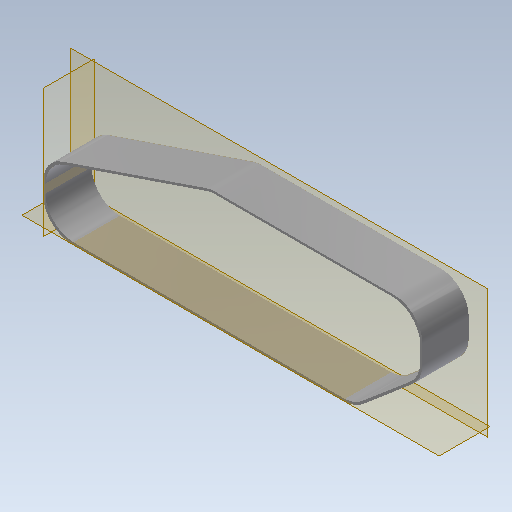
# Autodesk Inventor part: Rupsband
Saved by Autodesk Inventor 2021 (Build 250183000, 183)
## iProperties
Manager: PJ / DCS
Company: Emmaüs Bovenbouw Aalter
Created: 2020-11-19
Part Number: Rupsband
Material: S235
Catalog Web Link: http://emmausbovenbouw.op-weg.be/
Vendor: Emmaüsinstituut Bovenbouw Aalter
Document SubType Name: Modeling
Designer: Antho
Engineer: Declercq St.
Manufacturer: Standard
Standards Organization: Custom
Density: 7.86 g/cm^3
Appearance: Steel
Title: Algemene titel
Subject: Specifieke titel
Author: Antho
Keywords: Ruwe Ø xxxxx
Comments: Opmerking
Autodesk Inventor part; units mm, degrees
sketch "Sketch3" plane through (0, 0, 0) normal (0, 0, 1) x (1, 0, 0)
  line L0 (0, 0) -> (0, 51)
  line L1 (0, 51) -> (150, 51)
  line L2 (150, 51) -> (150, 102)
  line L3 (150, 102) -> (340, 102)
  line L4 (340, 102) -> (340, 51)
  line L5 (340, 51) -> (280, 51)
  line L6 (280, 51) -> (280, 0)
  line L7 (280, 0) -> (0, 0)
  line L8 (0, 51) -> (150, 102)
  line L9 (280, 0) -> (340, 51)
  dimension "d9" = 51
  dimension "d10" = 150
  dimension "d11" = 51
  dimension "d12" = 190
  dimension "d13" = 51
  dimension "d14" = 60
  constraints: 20 end point, 5 perpendicular, 2 point on line, 1 vertical
  measures "d9" distance of L0.start L0.end
  measures "d10" distance of L0.end L1.end
  measures "d11" distance of L1.end L2.end
  measures "d12" distance of L2.end L3.end
  measures "d13" distance of L3.end L4.end
  measures "d14" distance of L4.end L5.end
sketch "Sketch4" plane through (0, 0, 0) normal (1, 0, 0) x (0, 1, 0)
  line L0 (0, 0) -> (-2, 0)
  line L1 (-2, 0) -> (-2, 42)
  line L2 (-2, 42) -> (0, 42)
  line L3 (0, 42) -> (0, 0)
  dimension "d15" = 2
  dimension "d16" = 42
  constraints: 8 end point, 2 parallel, 1 horizontal, 1 perpendicular
  measures "d15" distance of L1.end L2.end
  measures "d16" distance of L0.end L1.end
sweep "Sweep2" add profiles "Sketch4" path "Sketch3" path curves L7 L9 L4 L3 L8 L0
fillet "Fillet1" radius 25.5 12 edges at (0, 51, 21) (-2, 52.4324, 21) (150, 102, 21) (149.6693, 104, 21) (-2, -2, 21) (0, 0, 21) (342, 104, 21) (340, 102, 21) (342, 50.0751, 21) (340, 51, 21) (280.7352, -2, 21) (280, 0, 21)
body "Solid2"
